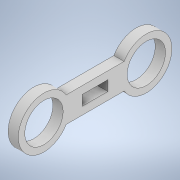
# Autodesk Inventor part: соединение пушек
Saved by Autodesk Inventor 2020.1 (Build 241239000, 239)
## iProperties
Created: 2022-03-19
Part Number: соединение пушек
Material: Типовые
Document SubType Name: Modeling
Designer: User
Density: 1 g/cm^3
Appearance: По умолчанию
Author: User
Autodesk Inventor part; units mm, degrees
ref_plane "YZ Plane" through (0, 0, 0) normal (1, 0, 0) x (0, 1, 0)
ref_plane "XZ Plane" through (0, 0, 0) normal (0, 1, 0) x (-1, 0, 0)
ref_plane "XY Plane" through (0, 0, 0) normal (0, 0, 1) x (1, 0, 0)
sketch "Эскиз1" plane through (0, 0, 0) normal (1, 0, 0) x (0, 1, 0)
  line L0 (0, 0) -> (10, 0)
  line L1 (10, 0) -> (10, 40)
  line L2 (10, 40) -> (0, 40)
  line L3 (0, 40) -> (0, 0)
  arc A0 (10, 40) -> (0, 40) centre (5, 40) ccw
  arc A1 (0, 0) -> (10, 0) centre (5, 0) ccw
  circle A2 centre (5, 40) radius 7.5
  circle A3 centre (5, 0) radius 7.5
  line L4 (0, 20) -> (10, 20)
  line L5 (0, 25) -> (-20, 25)
  line L6 (-20, 25) -> (-20, 15)
  line L7 (-20, 15) -> (0, 15)
  line L8 (0, 15) -> (0, 25)
  line L9 (7, 25) -> (3, 25)
  line L10 (3, 25) -> (3, 15)
  line L11 (3, 15) -> (7, 15)
  line L12 (7, 15) -> (7, 25)
  circle A4 centre (5, 40) radius 10
  circle A5 centre (5, 0) radius 10
  point P0 (0, 15)
  point P1 (0, 8.6603)
  point P2 (10, 8.6603)
  point P3 (10, 5.5902)
  point P4 (0, 5.5902)
  point P5 (10, 31.3397)
  point P6 (0, 31.3397)
  point P7 (0, 34.4098)
  point P8 (10, 34.4098)
  dimension "d0" = 40
  dimension "d1" = 10
  dimension "d2" = 15
  dimension "d3" = 15
  dimension "d6" = 10
  dimension "d7" = 20
  dimension "d8" = 10
  dimension "d9" = 20
  dimension "d10" = 20
  constraints: 26 end point, 6 centre point, 6 parallel, 4 coincident, 4 midpoint, 4 point on circle, 3 horizontal, 3 perpendicular, 1 point on line, 2 other
  measures "d0" distance of L0.end L1.end
  measures "d1" distance of L0.start L0.end
  measures "d2" diameter of A2
  measures "d3" diameter of A3
  measures "d6" distance of L5.end L6.end
  measures "d7" distance of L6.end L7.end
  measures "d8" distance of L11.end L9.start
  measures "d9" diameter of A4
  measures "d10" diameter of A5
extrude "Выдавливание1" add sketch "Эскиз1" along normal blind 4 contours A3 L1 A5 L3 | L3 A5 L1 A3 | L3 L4 L10 L11 L12 L1 A5 | L4 L12 L9 L10 L3 A4 L1 | A4 L3 A2 L1 | L1 A2 L3 A4
